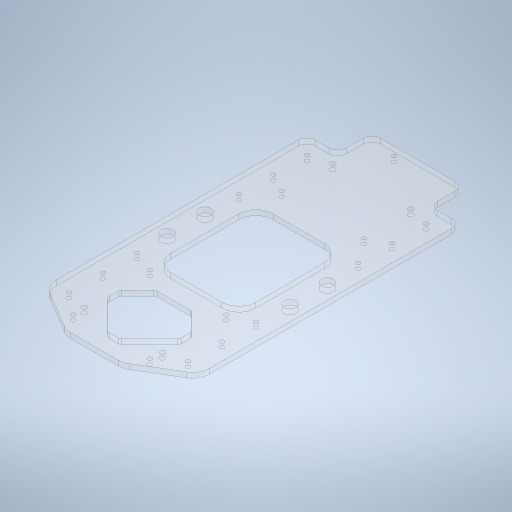
# Autodesk Inventor part: ElectronicsAntennaPlateV01
Saved by Autodesk Inventor 2023 (Build 270158000, 158)
## iProperties
Created: 2022-11-08
Part Number: ElectronicsAntennaPlateV01
Material: Polycarbonate, Clear
Document SubType Name: Modeling
Designer: Administrator
Density: 1.2 g/cm^3
Appearance: Polycarbonate - Clear
Author: Administrator
Autodesk Inventor part; units mm, degrees
ref_plane "YZ Plane" through (0, 0, 0) normal (1, 0, 0) x (0, 1, 0)
ref_plane "XZ Plane" through (0, 0, 0) normal (0, 1, 0) x (-1, 0, 0)
ref_plane "XY Plane" through (0, 0, 0) normal (0, 0, 1) x (1, 0, 0)
sketch "Sketch1" plane through (0, 0, 0) normal (0, 1, 0) x (-1, 0, 0)
  line L0 (10, 0) -> (80, 0)
  line L1 (90, -32.6619) -> (90, -167.3381)
  line L2 (67, -200) -> (23, -200)
  line L3 (0, -167.3381) -> (0, -32.6619)
  line L4 (22, -27) -> (68, -27) construction
  line L5 (68, -27) -> (68, -173) construction
  line L6 (68, -173) -> (22, -173) construction
  line L7 (22, -173) -> (22, -27) construction
  circle A0 centre (68, -27) radius 1.5
  circle A1 centre (68, -173) radius 1.5
  circle A2 centre (22, -173) radius 1.5
  circle A3 centre (22, -27) radius 1.5
  line L8 (30, -70) -> (60, -70)
  line L9 (70, -80) -> (70, -120)
  line L10 (60, -130) -> (30, -130)
  line L11 (20, -120) -> (20, -80)
  arc A4 (70, -80) -> (60, -70) centre (60, -80) ccw
  arc A5 (60, -130) -> (70, -120) centre (60, -120) ccw
  arc A6 (20, -120) -> (30, -130) centre (30, -120) ccw
  arc A7 (30, -70) -> (20, -80) centre (30, -80) ccw
  arc A8 (90, -10) -> (80, 0) centre (80, -10) ccw
  arc A9 (0, -190) -> (10, -200) centre (10, -190) ccw
  arc A10 (80, -200) -> (90, -190) centre (80, -190) ccw
  arc A11 (10, 0) -> (0, -10) centre (10, -10) ccw
  circle A12 centre (80, -10) radius 1.25
  circle A13 centre (80, -30) radius 1.25
  circle A14 centre (80, -50) radius 1.25
  circle A15 centre (80, -70) radius 1.25
  circle A16 centre (80, -90) radius 1.25
  circle A17 centre (80, -110) radius 1.25
  circle A18 centre (80, -130) radius 1.25
  circle A19 centre (80, -150) radius 1.25
  circle A20 centre (80, -170) radius 1.25
  circle A21 centre (80, -190) radius 1.25
  circle A22 centre (10, -10) radius 1.25
  circle A23 centre (10, -30) radius 1.25
  circle A24 centre (10, -50) radius 1.25
  circle A25 centre (10, -70) radius 1.25
  circle A26 centre (10, -90) radius 1.25
  circle A27 centre (10, -110) radius 1.25
  circle A28 centre (10, -130) radius 1.25
  circle A29 centre (10, -150) radius 1.25
  circle A30 centre (10, -170) radius 1.25
  circle A31 centre (10, -190) radius 1.25
  circle A32 centre (81, -111) radius 3.5
  circle A33 centre (81.25, -89) radius 3.5
  circle A34 centre (9, -111) radius 3.5
  circle A35 centre (9, -89) radius 3.5
  line L12 (85.145, -24.087) -> (64.0418, -11.4251)
  line L13 (4.855, -24.087) -> (25.9582, -11.4251)
  arc A36 (90, -32.6619) -> (85.145, -24.087) centre (80, -32.6619) ccw
  arc A37 (4.855, -24.087) -> (0, -32.6619) centre (10, -32.6619) ccw
  circle A38 centre (67.5, -65) radius 1.25
  circle A39 centre (22.5, -65) radius 1.25
  line L14 (-15, -70) -> (15, -70)
  circle A40 centre (67.5, -20) radius 1.25
  line L15 (30, -25) -> (60, -25)
  circle A41 centre (22.5, -20) radius 1.25
  line L16 (-15, -25) -> (15, -25)
  line L17 (58.8968, -10) -> (31.1032, -10)
  arc A42 (64.0418, -11.4251) -> (58.8968, -10) centre (58.8968, -20) ccw
  arc A43 (31.1032, -10) -> (25.9582, -11.4251) centre (31.1032, -20) ccw
  line L18 (45, -25) -> (45, -65)
  line L19 (45, -65) -> (45, -45)
  line L20 (67.5, -65) -> (22.5, -20) construction
  line L21 (67.5, -20) -> (22.5, -65) construction
  line L22 (65.6274, -46.6213) -> (56.1924, -56.0563)
  line L23 (33.8076, -56.0563) -> (24.3726, -46.6213)
  line L24 (24.3726, -38.3787) -> (40.8787, -21.8726)
  line L25 (49.1213, -21.8726) -> (65.6274, -38.3787)
  line L26 (69.7487, -42.5) -> (20.2513, -42.5) construction
  line L27 (45, -67.2487) -> (45, -17.7513) construction
  line L28 (54.7782, -56.6421) -> (35.2218, -56.6421)
  line L29 (66.2132, -45.2071) -> (66.2132, -39.7929)
  line L30 (23.7868, -45.2071) -> (23.7868, -39.7929)
  line L31 (47.7071, -21.2868) -> (42.2929, -21.2868)
  arc A44 (54.7782, -56.6421) -> (56.1924, -56.0563) centre (54.7782, -54.6421) ccw
  arc A45 (65.6274, -46.6213) -> (66.2132, -45.2071) centre (64.2132, -45.2071) ccw
  arc A46 (66.2132, -39.7929) -> (65.6274, -38.3787) centre (64.2132, -39.7929) ccw
  arc A47 (49.1213, -21.8726) -> (47.7071, -21.2868) centre (47.7071, -23.2868) ccw
  arc A48 (42.2929, -21.2868) -> (40.8787, -21.8726) centre (42.2929, -23.2868) ccw
  arc A49 (24.3726, -38.3787) -> (23.7868, -39.7929) centre (25.7868, -39.7929) ccw
  arc A50 (23.7868, -45.2071) -> (24.3726, -46.6213) centre (25.7868, -45.2071) ccw
  arc A51 (33.8076, -56.0563) -> (35.2218, -56.6421) centre (35.2218, -54.6421) ccw
  line L32 (90, -200) -> (72, -200) construction
  line L33 (72, -195) -> (72, -185)
  line L34 (77, -180) -> (85, -180)
  line L35 (90, -175) -> (90, -167.3381)
  line L36 (0, -200) -> (18, -200) construction
  line L37 (18, -195) -> (18, -185)
  line L38 (13, -180) -> (5, -180)
  line L39 (0, -175) -> (0, -167.3381)
  arc A52 (77, -180) -> (72, -185) centre (77, -185) ccw
  arc A53 (85, -180) -> (90, -175) centre (85, -175) ccw
  arc A54 (0, -175) -> (5, -180) centre (5, -175) ccw
  arc A55 (18, -185) -> (13, -180) centre (13, -185) ccw
  arc A56 (67, -200) -> (72, -195) centre (67, -195) ccw
  arc A57 (18, -195) -> (23, -200) centre (23, -195) ccw
  circle A58 centre (69.1385, -144.2) radius 1.25
  circle A59 centre (20.8615, -144.2) radius 1.25
  circle A60 centre (53.8985, -195) radius 1.25
  point P0 (0, 0)
  point P1 (90, 0)
  point P2 (70, -130)
  point P3 (70, -70)
  point P4 (20, -130)
  point P5 (45, 0)
  point P6 (45, -200)
  point P7 (25, -70)
  point P8 (70, -25)
  point P9 (25, -25)
  point P10 (45, -42.5)
  point P11 (55.6066, -56.6421)
  point P12 (34.3934, -56.6421)
  point P13 (66.2132, -46.0355)
  point P14 (66.2132, -38.9645)
  point P15 (23.7868, -46.0355)
  point P16 (23.7868, -38.9645)
  point P17 (48.5355, -21.2868)
  point P18 (41.4645, -21.2868)
  point P19 (72, -180)
  dimension "d0" = 90
  dimension "d1" = 200
  dimension "d2" = 46
  dimension "d4" = 22
  dimension "d5" = 27
  dimension "d6" = 3
  dimension "d7" = 3
  dimension "d8" = 3
  dimension "d9" = 3
  dimension "d10" = 50
  dimension "d11" = 60
  dimension "d12" = 20
  dimension "d13" = 70
  dimension "d14" = 10
  dimension "d15" = 10
  dimension "d16" = 2.5
  dimension "d19" = 20
  dimension "d24" = 2.5
  dimension "d27" = 20
  dimension "d34" = 7
  dimension "d35" = 7
  dimension "d36" = 7
  dimension "d37" = 7
  dimension "d38" = 72
  dimension "d39" = 22
  dimension "d40" = 9
  dimension "d41" = 89
  dimension "d42" = 22
  dimension "d43" = 72
  dimension "d46" = 10
  dimension "d48" = 2.5
  dimension "d51" = 45
  dimension "d54" = 45
  dimension "d57" = 22.5
  dimension "d58" = 5
  dimension "d59" = 10
  dimension "d60" = 35
  dimension "d61" = 35
  dimension "d62" = 15
  dimension "d63" = 15
  dimension "d64" = 5
  dimension "d65" = 5
  dimension "d66" = 5
  dimension "d67" = 5
  dimension "d68" = 5
  dimension "d69" = 5
  dimension "d70" = 2
  dimension "d71" = 18
  dimension "d72" = 20
  dimension "d73" = 18
  dimension "d74" = 5
  dimension "d75" = 5
  dimension "d76" = 2.5
  dimension "d77" = 2.5
  dimension "d78" = 0
  dimension "d79" = 48.277
  dimension "d81" = 20.8615
  dimension "d82" = 2.5
  dimension "d83" = 15.24
  dimension "d84" = 50.8
  dimension "d85" = 5
  constraints: 78 end point, 61 centre point, 52 point on circle, 49 point on line, 48 tangent, 19 equal radius, 9 perpendicular, 8 parallel, 6 coincident, 6 horizontal, 6 midpoint, 4 vertical, 1 collinear, 67 other
  measures "d0" distance of L32.start L36.start
  measures "d1" distance of point (90, 0) L32.start
  measures "d2" distance of L5.end L6.end
  measures "d4" distance between parallel lines of L1 L5
  measures "d6" diameter of A0
  measures "d7" diameter of A1
  measures "d8" diameter of A2
  measures "d9" diameter of A3
  measures "d10" distance of point (70, -130) point (20, -130)
  measures "d11" distance of point (70, -70) point (70, -130)
  measures "d12" distance between parallel lines of L3 L11
  measures "d13" distance between parallel lines of L0 L8
  measures "d14" radius of A4
  measures "d15" radius of A8
  measures "d16" diameter of A12
  measures "d19" distance of A12.centre A13.centre
  measures "d24" diameter of A22
  measures "d27" distance of A22.centre A23.centre
  measures "d34" diameter of A32
  measures "d35" diameter of A33
  measures "d36" diameter of A34
  measures "d37" diameter of A35
  measures "d38" distance of A34.centre A32.centre
  measures "d39" distance of A35.centre A34.centre
  measures "d40" distance from line of L3 A34.centre
  measures "d42" vertical distance of A34.centre A33.centre
  measures "d43" horizontal distance of A35.centre A32.centre
  measures "d46" radius of A36
  measures "d48" diameter of A38
  measures "d51" distance of L20.start L21.end
  measures "d54" distance of L20.start L21.start
  measures "d57" distance from line of L1 L20.start
  measures "d58" distance from line of L8 L20.start
  measures "d59" radius of A42
  measures "d60" distance of L26.start L27.start
  measures "d61" distance of L27.start L26.end
  measures "d62" distance of point (55.607, -56.642) L27.start
  measures "d63" distance of point (34.393, -56.642) L27.start
  measures "d64" distance of point (66.213, -46.036) L26.start
  measures "d65" distance of point (66.213, -38.964) L26.start
  measures "d66" distance of point (23.787, -46.036) L26.end
  measures "d67" distance of point (23.787, -38.964) L26.end
  measures "d68" distance of point (48.536, -21.287) L27.end
  measures "d69" distance of point (41.464, -21.287) L27.end
  measures "d70" radius of A44
  measures "d71" distance of L32.start L32.end
  measures "d72" distance of L32.end point (72, -180)
  measures "d73" distance of L36.start L36.end
  measures "d74" radius of A52
  measures "d75" radius of A56
  measures "d76" diameter of A58
  measures "d77" diameter of A59
  measures "d78" vertical distance of A59.centre A58.centre
  measures "d79" distance of A59.centre A58.centre
  measures "d81" distance from line of L3 A59.centre
  measures "d82" diameter of A60
  measures "d83" horizontal distance of A60.centre A58.centre
  measures "d84" vertical distance of A58.centre A60.centre
extrude "Extrusion2" add sketch "Sketch1" along normal blind 3 contours L1 L35 A53 L34 A52 L33 A56 L2 A57 L37 A55 L38 A54 L39 L3 A37 L13 A43 L17 A42 L12 A36
equation "\"d4\" = -0.5 * d2 + 0.5 * d0"
equation "\"d5\" = -0.5 * d3 + 0.5 * d1"
equation "\"d12\" = -0.5 * d10 + 0.5 * d0"
equation "\"d13\" = -0.5 * d11 + 0.5 * d1"
equation "\"d40\" = -0.5 * d38 + 0.5 * d0"
equation "\"d41\" = -0.5 * d39 + 0.5 * d1"
equation "\"d57\" = -0.5 * d51 + 0.5 * d0"
equation "\"d63\" = d62"
equation "\"d65\" = d64"
equation "\"d66\" = d64"
equation "\"d67\" = d66"
equation "\"d68\" = d64"
equation "\"d69\" = d68"
equation "\"d81\" = -0.5 * d79 + 0.5 * d0"
equation "\"d3\" = 146"
body "Solid2"
